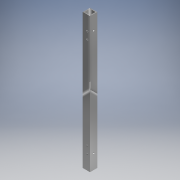
# Autodesk Inventor part: 15102898-16-P-0209
Saved by Autodesk Inventor 2017 (Build 210142000, 142)
## iProperties
Created: 2016-10-03
Part Number: 15102898-16-P-0209
Material: Aluminum 6061
Document SubType Name: Modeling
Designer: gus
Density: 2.7 g/cm^3
Appearance: Aluminum - Flat
Mass: 263.99 g
Surface Area: 626.612 cm^2
Volume: 97.774 cm^3
Author: gus
Autodesk Inventor part; units mm, degrees
ref_plane "YZ Plane" through (0, 0, 0) normal (1, 0, 0) x (0, 1, 0)
ref_plane "XZ Plane" through (0, 0, 0) normal (0, 1, 0) x (-1, 0, 0)
ref_plane "XY Plane" through (0, 0, 0) normal (0, 0, 1) x (1, 0, 0)
sketch "Sketch1" plane through (0, 0, 0) normal (0, 1, 0) x (-1, 0, 0)
  line L0 (0, 0) -> (25.4, 0)
  line L1 (25.4, 0) -> (25.4, -25.4)
  line L2 (25.4, -25.4) -> (0, -25.4)
  line L3 (0, -25.4) -> (0, 0)
  line L4 (22.225, -22.225) -> (22.225, -3.175)
  line L5 (22.225, -3.175) -> (3.175, -3.175)
  line L6 (3.175, -3.175) -> (3.175, -22.225)
  line L7 (3.175, -22.225) -> (22.225, -22.225)
  dimension "d0" = 25.4
  dimension "d1" = 25.4
  dimension "d2" = 3.175
  constraints: 16 end point, 4 parallel, 2 perpendicular, 1 horizontal, 3 other
  measures "d0" distance of L1.end L2.end
  measures "d1" distance of L0.end L1.end
  measures "d2" distance between parallel lines of L1 L4
extrude "Extrusion1" add sketch "Sketch1" along normal blind 476.25
sketch "Sketch2" plane through (0, 0, 0) normal (1, 0, 0) x (0, 0, -1)
  line L0 (0, 0) -> (0, 476.25) projected
  line L1 (25.4, 0) -> (0, 0) projected
  line L2 (0, 476.25) -> (25.4, 476.25) projected
  point P0 (12.7, 50.8)
  point P1 (12.7, 425.45)
  dimension "d6" = 12.7
  dimension "d9" = 12.7
  dimension "d10" = 50.8
  dimension "d12" = 50.8
  measures "d6" distance from line of L0 point (12.7, 425.45)
  measures "d9" distance from line of L0 point (12.7, 50.8)
  measures "d10" distance from line of L1 point (12.7, 50.8)
  measures "d12" distance from line of L2 point (12.7, 425.45)
hole "Hole1" at (0, 50.8, -12.7) at (0, 425.45, -12.7) direction (-1, 0, 0) diameter 6.35 end through all
sketch "Sketch3" plane through (0, 0, -25.4) normal (0, 0, -1) x (-1, 0, 0)
  line L0 (25.4, 0) -> (0, 0) projected
  line L1 (0, 476.25) -> (25.4, 476.25) projected
  line L2 (25.4, 0) -> (25.4, 476.25) projected
  point P0 (9.525, 50.8)
  point P1 (9.525, 425.45)
  point P2 (9.525, 400.05)
  point P3 (9.525, 76.2)
  dimension "d20" = 50.8
  dimension "d21" = 50.8
  dimension "d22" = 25.4
  dimension "d23" = 25.4
  dimension "d24" = 15.875
  dimension "d25" = 15.875
  dimension "d26" = 15.875
  dimension "d27" = 15.875
  measures "d20" distance from line of L0 point (9.525, 50.8)
  measures "d21" distance from line of L1 point (9.525, 425.45)
  measures "d22" distance of point (9.525, 425.45) point (9.525, 400.05)
  measures "d23" distance of point (9.525, 76.2) point (9.525, 50.8)
  measures "d24" distance from line of point (9.525, 50.8) L2
  measures "d25" distance from line of L2 point (9.525, 76.2)
  measures "d26" distance from line of L2 point (9.525, 400.05)
  measures "d27" distance from line of L2 point (9.525, 425.45)
hole "Hole2" at (-9.525, 50.8, -25.4) at (-9.525, 425.45, -25.4) at (-9.525, 400.05, -25.4) at (-9.525, 76.2, -25.4) direction (0, 0, 1) diameter 6.7469 end through all
body "Solid1"
